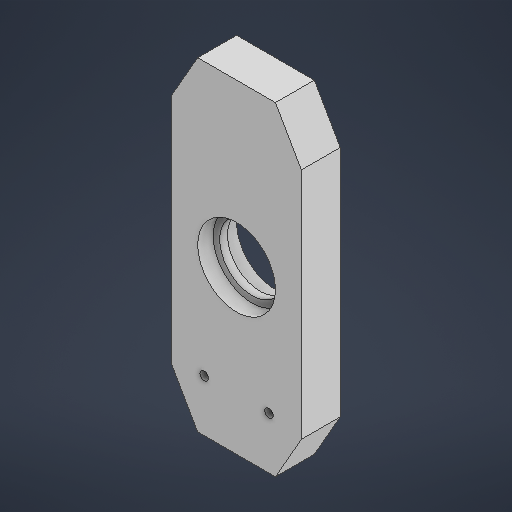
# Autodesk Inventor part: Suspension_Upright_V2
Saved by Autodesk Inventor 2026.1 (Build 301233000, 233)
## iProperties
Created: 2026-08-18
Part Number: Suspension_Upright_V2
Material: Generic
Document SubType Name: Modeling
Designer: share
Density: 1 g/cm^3
Appearance: Default
Author: share
Autodesk Inventor part; units mm, degrees
ref_plane "YZ Plane" through (0, 0, 0) normal (1, 0, 0) x (0, 1, 0)
ref_plane "XY Plane" through (0, 0, 0) normal (0, 0, 1) x (1, 0, 0)
ref_plane "Upper Pickup Plane" through (0, 110, 0) normal (0, 1, 0) x (-1, 0, 0)
ref_plane "Lower Pickup Plane" through (0, -110, 0) normal (0, 1, 0) x (-1, 0, 0)
sketch "Sketch1" plane through (0, 0, 0) normal (0, 0, 1) x (1, 0, 0)
  line L0 (-70, 0) -> (70, 0) construction
  line L1 (0, 175) -> (0, -175) construction
  line L2 (30, -125) -> (-30, -125)
  line L3 (-50, -90) -> (-50, 90)
  line L4 (-30, 125) -> (30, 125)
  line L5 (50, 90) -> (50, -90)
  line L6 (-30, 125) -> (-50, 90)
  line L7 (30, 125) -> (50, 90)
  line L8 (-50, 90) -> (50, 90) construction
  line L9 (-30, -125) -> (-50, -90)
  line L10 (30, -125) -> (50, -90)
  line L11 (-50, -90) -> (50, -90) construction
  line L12 (-50, 90) -> (-50, 125) construction
  line L13 (50, 90) -> (50, 125) construction
  line L14 (-30, 125) -> (-50, 125) construction
  line L15 (30, 125) -> (50, 125) construction
  line L16 (-50, -90) -> (-50, -125) construction
  line L17 (-30, -125) -> (-50, -125) construction
  line L18 (30, -125) -> (50, -125) construction
  line L19 (50, -90) -> (50, -125) construction
  point P0 (0, 0)
  point P1 (0, 110)
  point P2 (0, -110)
  dimension "d8" = 180
  dimension "d9" = 60
  dimension "d11" = 250
  dimension "d12" = 100
  constraints: 36 end point, 6 symmetric about line, 5 perpendicular, 4 horizontal, 2 parallel, 2 vertical, 2 other
  measures "d8" distance between parallel lines of L11 L8
  measures "d9" distance of L2.end L2.start
  measures "d11" distance between parallel lines of L2 L4
  measures "d12" distance between parallel lines of L5 L3
extrude "Main Body" add sketch "Sketch1" along normal mid plane 30
sketch "Sketch2" plane through (0, 0, 15) normal (0, 0, 1) x (1, 0, 0)
  circle A0 centre (0, 0) radius 25
  dimension "d13" = 50
  constraints: 1 centre point, 1 coincident
  measures "d13" diameter of A0
extrude "Axle Bore" cut sketch "Sketch2" against normal through all
sketch "Sketch3" plane through (0, 0, 15) normal (0, 0, 1) x (1, 0, 0)
  circle A0 centre (0, 0) radius 30
  circle A1 centre (0, 0) radius 25 projected
  dimension "d16" = 60
  constraints: 1 centre point, 1 coincident
  measures "d16" diameter of A0
extrude "Front Side Bearing Pocket" cut sketch "Sketch3" against normal blind 12
sketch "Sketch4" plane through (0, 0, -15) normal (0, 0, -1) x (-1, 0, 0)
  circle A0 centre (0, 0) radius 30 projected
  circle A1 centre (0, 0) radius 25 projected
extrude "Back Side Bearing Pocket" cut sketch "Sketch4" against normal blind 12
sketch "Sketch5" plane through (0, 0, 15) normal (0, 0, 1) x (1, 0, 0)
  line L0 (-50, 90) -> (-50, -90) projected
  line L1 (-50, -85) -> (50, -85) construction
  line L2 (50, -90) -> (50, 90) projected
  line L3 (0, 175) -> (0, -175) construction
  point P0 (0, 0)
  point P1 (0, -110)
  point P2 (-25, -85)
  point P3 (25, -85)
  dimension "d23" = 25
  dimension "d24" = 50
  constraints: 4 point on line, 2 end point, 1 horizontal, 1 symmetric about line
  measures "d23" distance from line of L1 point (0, -110)
  measures "d24" distance of point (25, -85) point (-25, -85)
hole "Hole1" at (-25, -85, 15) at (25, -85, 15) direction (0, 0, -1) diameter 6.647 depth 30 thread size "M8x1.25" class "6H" standard "ANSI Metric M Profile"
equation "\"d4\" = Upright_Thickness"
equation "\"d13\" = Axle_Bore_Diameter"
equation "\"d16\" = Wheel_Bearing_Bore_Diameter"
equation "\"d17\" = Wheel_Bearing_Thickness"
equation "\"d19\" = Wheel_Bearing_Thickness"
equation "\"d23\" = arm_z"
equation "\"d26\" = Upright_Thickness"
equation "\"Upright_Thickness\" = 30"
equation "\"Axle_Bore_Diameter\" = 50"
equation "\"Wheel_Bearing_Bore_Diameter\" = 60"
equation "\"Wheel_Bearing_Thickness\" = 12"
equation "\"arm_z\" = 25"
body "Solid1"
